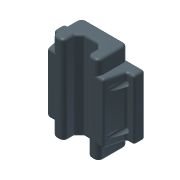
# Autodesk Inventor part: bLOCK
Saved by Autodesk Inventor 2014 (Build 180170000, 170)
## iProperties
Created: 2014-08-09
Part Number: bLOCK
Material: Generic
Document SubType Name: Modeling
Designer: Peele
Density: 1 g/cm^3
Appearance: Lead
Author: Peele
Autodesk Inventor part; units mm, degrees
ref_plane "YZ Plane" through (0, 0, 0) normal (1, 0, 0) x (0, 1, 0)
ref_plane "XZ Plane" through (0, 0, 0) normal (0, 1, 0) x (-1, 0, 0)
ref_plane "XY Plane" through (0, 0, 0) normal (0, 0, 1) x (1, 0, 0)
sketch "Sketch1" plane through (0, 0, 0) normal (0, 0, 1) x (1, 0, 0)
  line L0 (-15, -9.5) -> (15, -9.5)
  line L1 (15, -9.5) -> (15, 9.5)
  line L2 (15, 9.5) -> (-15, 9.5)
  line L3 (-15, 9.5) -> (-15, -9.5)
  line L4 (-15, -9.5) -> (15, 9.5) construction
  line L5 (15, -9.5) -> (-15, 9.5) construction
  line L6 (-7.5, 0.5) -> (7.5, 0.5)
  line L7 (7.5, 0.5) -> (7.5, -9.5)
  line L8 (7.5, -9.5) -> (-7.5, -9.5)
  line L9 (-7.5, -9.5) -> (-7.5, 0.5)
  line L10 (-7.5, 0.5) -> (7.5, -9.5) construction
  line L11 (7.5, 0.5) -> (-7.5, -9.5) construction
  line L12 (0, -4.5) -> (0, 0)
  dimension "d0" = 15
  dimension "d1" = 19
  dimension "d2" = 30
  dimension "d3" = 10
  constraints: 26 end point, 5 midpoint, 5 parallel, 2 horizontal, 2 perpendicular, 1 coincident, 1 point on line
  measures "d0" distance of L7.end L8.end
  measures "d1" distance of L2.end L0.start
  measures "d2" distance of L1.end L2.end
  measures "d3" distance of L6.end L7.end
extrude "Extrusion1" add sketch "Sketch1" along normal mid plane 56.9 contours L3 L2 L1 L0 L7 L6 L9
chamfer "Chamfer1" distance 3 angle 45 2 edges at (-7.5, 0.5, 0) (7.5, 0.5, 0)
fillet "Fillet1" radius 3 6 edges at (-15, -9.5, 0) (-7.5, -9.5, 0) (7.5, -9.5, 0) (15, -9.5, 0) (15, 9.5, 0) (-15, 9.5, 0)
fillet "Fillet2" radius 1.5 32 edges at (-14.1213, 8.6213, 28.45) (-15, 0, 28.45) (-14.1213, -8.6213, 28.45) (-11.25, -9.5, 28.45) (-8.3787, -8.6213, 28.45) (-7.5, -4.5, 28.45) (14.1213, 8.6213, 28.45) (15, 0, 28.45) (14.1213, -8.6213, 28.45) (11.25, -9.5, 28.45) (8.3787, -8.6213, 28.45) (7.5, -4.5, 28.45) (0, 9.5, 28.45) (6, -1, 28.45) (0, 0.5, 28.45) (-6, -1, 28.45) (-14.1213, 8.6213, -28.45) (0, 9.5, -28.45) (14.1213, 8.6213, -28.45) (15, 0, -28.45) (14.1213, -8.6213, -28.45) (11.25, -9.5, -28.45) (8.3787, -8.6213, -28.45) (7.5, -4.5, -28.45) (-14.1213, -8.6213, -28.45) (-11.25, -9.5, -28.45) (-8.3787, -8.6213, -28.45) (-7.5, -4.5, -28.45) (-15, 0, -28.45) (-6, -1, -28.45) (0, 0.5, -28.45) (6, -1, -28.45)
sketch "Sketch2" plane through (0, 0, 0) normal (0, 0, 1) x (1, 0, 0)
  line L0 (-26, 9.5) -> (-26, 2.5)
  line L1 (-26, 2.5) -> (-21, 2.5)
  line L2 (-21, 2.5) -> (-18, -9.5)
  line L3 (-18, -9.5) -> (-12, -9.5)
  line L4 (-12, -9.5) -> (-12, 9.5)
  line L5 (-12, 9.5) -> (-26, 9.5)
  line L6 (-12, 9.5) -> (12, 9.5) projected
  line L7 (-10.5, -9.5) -> (-12, -9.5) projected
  point P0 (0, 0)
  dimension "d11" = 7
  dimension "d12" = 26
  dimension "d13" = 6
  dimension "d14" = 5
  constraints: 12 end point, 2 collinear, 2 vertical, 1 horizontal, 1 parallel, 1 perpendicular
  measures "d11" distance of L0.start L0.end
  measures "d12" distance from line of point (0, 0) L0
  measures "d13" distance of L2.end L3.end
  measures "d14" distance of L0.end L1.end
extrude "Extrusion2" add sketch "Sketch2" along normal mid plane 38.7
fillet "Fillet3" radius 1.5 14 edges at (-26, 9.5, 0) (-26, 2.5, 0) (-21, 2.5, 0) (-18, -9.5, 0) (-19.5, -3.5, 19.35) (-23.5, 2.5, 19.35) (-15, -9.5, 19.35) (-19, 9.5, 19.35) (-26, 6, 19.35) (-19.5, -3.5, -19.35) (-15, -9.5, -19.35) (-23.5, 2.5, -19.35) (-26, 6, -19.35) (-19, 9.5, -19.35)
mirror "Mirror1" about plane through (0, 0, 0) normal (1, 0, 0) of "Fillet3", "Extrusion2"
sketch "Sketch3" plane through (-12, 9.5, -26.95) normal (0, 1, 0) x (1, 0, 0)
  line L0 (-8.5, -39.95) -> (32.5, -39.95) construction
  line L1 (32.5, -39.95) -> (32.5, -13.95) construction
  line L2 (32.5, -13.95) -> (-8.5, -13.95) construction
  line L3 (-8.5, -13.95) -> (-8.5, -39.95) construction
  line L4 (-8.5, -39.95) -> (32.5, -13.95) construction
  line L5 (32.5, -39.95) -> (-8.5, -13.95) construction
  circle A0 centre (-8.5, -13.95) radius 2
  circle A1 centre (32.5, -13.95) radius 2
  circle A2 centre (32.5, -39.95) radius 2
  circle A3 centre (-8.5, -39.95) radius 2
  point P0 (12, -26.95)
  dimension "d18" = 26
  dimension "d19" = 41
  dimension "d20" = 4
  constraints: 12 end point, 4 centre point, 4 coincident, 3 equal radius, 2 midpoint, 2 parallel, 1 horizontal, 1 perpendicular
  measures "d18" distance of L0.end L1.end
  measures "d19" distance of L0.start L0.end
  measures "d20" diameter of A2
extrude "Extrusion3" cut sketch "Sketch3" against normal through all
ref_plane "Work Plane1" through (0, 0, 0) normal (1, 0, 0) x (0, 1, 0)
body "Solid1"
